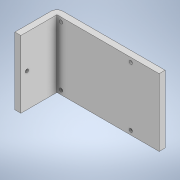
# Autodesk Inventor part: Pi4Bracket
Saved by Autodesk Inventor 2022 (Build 260153000, 153)
## iProperties
Created: 2022-01-26
Part Number: Pi4Bracket
Material: Generic
Document SubType Name: Modeling
Designer: junji
Density: 1 g/cm^3
Appearance: Default
Author: junji
Autodesk Inventor part; units mm, degrees
ref_plane "YZ Plane" through (0, 0, 0) normal (1, 0, 0) x (0, 1, 0)
ref_plane "XZ Plane" through (0, 0, 0) normal (0, 1, 0) x (-1, 0, 0)
ref_plane "XY Plane" through (0, 0, 0) normal (0, 0, 1) x (1, 0, 0)
sketch "Sketch1" plane through (0, 0, 0) normal (0, 0, 1) x (1, 0, 0)
  line L0 (-45, 28) -> (45, 28)
  line L1 (45, 28) -> (45, -28)
  line L2 (45, -28) -> (-45, -28)
  line L3 (-45, -28) -> (-45, 28)
  line L4 (-45, 28) -> (45, -28) construction
  line L5 (45, 28) -> (-45, -28) construction
  line L6 (-40, -28) -> (-40, 28)
  circle A0 centre (-36.5, 24.5) radius 1.35
  line L7 (-10.2595, 0) -> (11.3926, 0)
  line L8 (-36.5, 24.5) -> (-7.5, 24.5)
  line L9 (-7.5, 24.5) -> (-7.5, 0)
  circle A1 centre (21.5, 24.5) radius 1.35
  circle A2 centre (-36.5, -24.5) radius 1.35
  circle A3 centre (21.5, -24.5) radius 1.35
  point P0 (0, 0)
  dimension "d0" = 90
  dimension "d1" = 56
  dimension "d4" = 5
  dimension "d5" = 2.7
  dimension "d6" = 3.5
  dimension "d7" = 3.5
  dimension "d8" = 29
  dimension "d9" = 49
  constraints: 20 end point, 4 centre point, 3 horizontal, 3 perpendicular, 3 point on line, 2 midpoint, 2 parallel, 2 symmetric about line, 3 other
  measures "d0" distance of L1.end L2.end
  measures "d1" distance of L0.end L1.end
  measures "d4" distance of L6.start L2.end
  measures "d5" diameter of A0
  measures "d6" distance from line of L0 L8.start
  measures "d7" distance from line of L6 L8.start
  measures "d8" distance of L8.start L8.end
  measures "d9" distance of A3.centre A1.centre
extrude "Extrusion1" add sketch "Sketch1" along normal blind 5 contours L0 L1 L2 L6
sketch "Sketch4" plane through (-40, -28, 0) normal (-1, 0, 0) x (0, 0, 1)
  line L0 (0, 0) -> (5, 0) projected
  line L1 (0, 0) -> (35, 0)
  line L2 (35, 0) -> (35, 56)
  line L3 (35, 56) -> (0, 56)
  line L4 (0, 56) -> (0, 0)
  circle A0 centre (30, 28) radius 1.35
  point P0 (0, 28)
  dimension "d19" = 35
  dimension "d20" = 2.7
  dimension "d21" = 5
  dimension "d22" = 28
  dimension "d25" = 56
  constraints: 8 end point, 2 parallel, 1 centre point, 1 horizontal, 1 perpendicular
  measures "d19" distance of L3.end L2.end
  measures "d20" diameter of A0
  measures "d21" distance from line of L2 A0.centre
  measures "d22" distance from line of L1 A0.centre
  measures "d25" distance of L1.end L2.end
extrude "Extrusion3" add sketch "Sketch4" along normal blind 5
fillet "Fillet1" radius 5 1 edges at (-45, 0, 0)
body "Solid1"
